Autodesk Fusion 360 part; units mm, degrees
note: some values were not read from the file. Set by a fixed rule: which sketch regions a step uses.
(part 8 of 10)
  spline S44 degree 5 poles (-2.127, 15.858) (-2.1276, 15.856) (-2.1289, 15.8519) (-2.1307, 15.8458) (-2.1332, 15.8377) (-2.1363, 15.8275) (-2.1394, 15.8174) (-2.1424, 15.8074) (-2.1454, 15.7973) (-2.1484, 15.7872) (-2.1514, 15.7772) (-2.1543, 15.7672) (-2.1573, 15.7572) (-2.1602, 15.7473) (-2.163, 15.7373) (-2.1659, 15.7274) (-2.1687, 15.7175) (-2.1715, 15.7076) (-2.1743, 15.6978) (-2.1771, 15.6879) (-2.1798, 15.6781) (-2.1825, 15.6683) (-2.1852, 15.6585) (-2.1879, 15.6488) (-2.1905, 15.6391) (-2.1931, 15.6294) (-2.1957, 15.6197) (-2.1983, 15.61) (-2.2008, 15.6004) (-2.2034, 15.5908) (-2.2059, 15.5812) (-2.2084, 15.5716) (-2.2108, 15.5621) (-2.2133, 15.5526) (-2.2157, 15.5431) (-2.2181, 15.5336) (-2.2204, 15.5241) (-2.2228, 15.5147) (-2.2251, 15.5053) (-2.2274, 15.4959) (-2.2297, 15.4866) (-2.232, 15.4772) (-2.2342, 15.4679) (-2.2364, 15.4586) (-2.2386, 15.4494) (-2.2408, 15.4402) (-2.2429, 15.431) (-2.2451, 15.4218) (-2.2472, 15.4126) (-2.2492, 15.4035) (-2.2513, 15.3944) (-2.2533, 15.3853) (-2.2554, 15.3762) (-2.2574, 15.3672) (-2.2593, 15.3582) (-2.2613, 15.3492) (-2.2632, 15.3403) (-2.2651, 15.3313) (-2.267, 15.3224) (-2.2689, 15.3136) (-2.2707, 15.3047) (-2.2726, 15.2959) (-2.2744, 15.2871) (-2.2761, 15.2784) (-2.2779, 15.2696) (-2.2796, 15.2609) (-2.2814, 15.2522) (-2.2831, 15.2436) (-2.2847, 15.2349) (-2.2864, 15.2263) (-2.288, 15.2178) (-2.2897, 15.2092) (-2.2913, 15.2007) (-2.2928, 15.1922) (-2.2944, 15.1838) (-2.2959, 15.1753) (-2.2974, 15.1669) (-2.2989, 15.1586) (-2.3004, 15.1502) (-2.3019, 15.1419) (-2.3033, 15.1336) (-2.3047, 15.1254) (-2.3061, 15.1172) (-2.3075, 15.109) (-2.3088, 15.1008) (-2.3102, 15.0927) (-2.3115, 15.0846) (-2.3128, 15.0765) (-2.3141, 15.0685) (-2.3153, 15.0605) (-2.3166, 15.0525) (-2.3178, 15.0445) (-2.319, 15.0366) (-2.3202, 15.0288) (-2.3213, 15.0209) (-2.3225, 15.0131) (-2.3236, 15.0053) (-2.3247, 14.9975) (-2.3258, 14.9898) (-2.3269, 14.9821) (-2.3279, 14.9745) (-2.329, 14.9669) (-2.33, 14.9593) (-2.331, 14.9517) (-2.332, 14.9442) (-2.3329, 14.9367) (-2.3339, 14.9292) (-2.3348, 14.9218) (-2.3357, 14.9144) (-2.3366, 14.9071) (-2.3375, 14.8998) (-2.3383, 14.8925) (-2.3391, 14.8852) (-2.34, 14.878) (-2.3408, 14.8708) (-2.3416, 14.8637) (-2.3423, 14.8566) (-2.3431, 14.8495) (-2.3438, 14.8425) (-2.3445, 14.8355) (-2.3452, 14.8285) (-2.3459, 14.8216) (-2.3466, 14.8147) (-2.3472, 14.8079) (-2.3479, 14.801) (-2.3485, 14.7943) (-2.3491, 14.7875) (-2.3497, 14.7808) (-2.3503, 14.7742) (-2.3508, 14.7675) (-2.3513, 14.7609) (-2.3519, 14.7544) (-2.3524, 14.7479) (-2.3529, 14.7414) (-2.3534, 14.735) (-2.3538, 14.7286) (-2.3543, 14.7222) (-2.3547, 14.7159) (-2.3551, 14.7097) (-2.3555, 14.7034) (-2.3559, 14.6972) (-2.3563, 14.6911) (-2.3567, 14.685) (-2.357, 14.6789) (-2.3574, 14.6729) (-2.3577, 14.6669) (-2.358, 14.6609) (-2.3583, 14.655) (-2.3586, 14.6492) (-2.3588, 14.6434) (-2.3591, 14.6376) (-2.3593, 14.6319) (-2.3596, 14.6262) (-2.3598, 14.6205) (-2.36, 14.6149) (-2.3602, 14.6094) (-2.3603, 14.6039) (-2.3605, 14.5984) (-2.3607, 14.593) (-2.3608, 14.5876) (-2.3609, 14.5823) (-2.3611, 14.577) (-2.3612, 14.5718) (-2.3613, 14.5666) (-2.3614, 14.5614) (-2.3614, 14.5563) (-2.3615, 14.5513) (-2.3616, 14.5463) (-2.3616, 14.5413) (-2.3616, 14.5364) (-2.3617, 14.5315) (-2.3617, 14.5267) (-2.3617, 14.5219) (-2.3617, 14.5172) (-2.3616, 14.5126) (-2.3616, 14.5079) (-2.3616, 14.5034) (-2.3616, 14.4989) (-2.3615, 14.4944) (-2.3614, 14.49) (-2.3614, 14.4856) (-2.3613, 14.4813) (-2.3612, 14.477) (-2.3611, 14.4728) (-2.361, 14.4687) (-2.3609, 14.4646) (-2.3608, 14.4605) (-2.3607, 14.4565) (-2.3606, 14.4526) (-2.3604, 14.4487) (-2.3603, 14.4449) (-2.3602, 14.4411) (-2.36, 14.4374) (-2.3599, 14.4337) (-2.3597, 14.4301) (-2.3595, 14.4265) (-2.3594, 14.423) (-2.3592, 14.4196) (-2.359, 14.4162) (-2.3588, 14.4129) (-2.3586, 14.4096) (-2.3584, 14.4064) (-2.3583, 14.4032) (-2.3581, 14.4001) (-2.3579, 14.3971) (-2.3577, 14.3941) (-2.3575, 14.3912) (-2.3572, 14.3884) (-2.357, 14.3856) (-2.3568, 14.3829) (-2.3566, 14.3802) (-2.3564, 14.3776) (-2.3562, 14.3751) (-2.356, 14.3726) (-2.3558, 14.3702) (-2.3556, 14.3679) (-2.3554, 14.3656) (-2.3551, 14.3634) (-2.3549, 14.3612) (-2.3547, 14.3591) (-2.3545, 14.3571) (-2.3543, 14.3552) (-2.3541, 14.3533) (-2.3539, 14.3515) (-2.3537, 14.3498) (-2.3536, 14.3481) (-2.3534, 14.3465) (-2.3532, 14.345) (-2.353, 14.3436) (-2.3529, 14.3422) (-2.3527, 14.3409) (-2.3525, 14.3397) (-2.3524, 14.3385) (-2.3522, 14.3374) (-2.3521, 14.3364) (-2.352, 14.3355) (-2.3519, 14.3346) (-2.3518, 14.3339) (-2.3517, 14.3332) (-2.3516, 14.3326) (-2.3515, 14.332) (-2.3514, 14.3317) (-2.3514, 14.3314) (-2.3514, 14.3313) (-2.3514, 14.3312) knots -1 -1 -1 -1 -1 -1 -0.99583333 -0.99166667 -0.9875 -0.98333333 -0.97916667 -0.975 -0.97083333 -0.96666667 -0.9625 -0.95833333 -0.95416667 -0.95 -0.94583333 -0.94166667 -0.9375 -0.93333333 -0.92916667 -0.925 -0.92083333 -0.91666667 -0.9125 -0.90833333 -0.90416667 -0.9 -0.89583333 -0.89166667 -0.8875 -0.88333333 -0.87916667 -0.875 -0.87083333 -0.86666667 -0.8625 -0.85833333 -0.85416667 -0.85 -0.84583333 -0.84166667 -0.8375 -0.83333333 -0.82916667 -0.825 -0.82083333 -0.81666667 -0.8125 -0.80833333 -0.80416667 -0.8 -0.79583333 -0.79166667 -0.7875 -0.78333333 -0.77916667 -0.775 -0.77083333 -0.76666667 -0.7625 -0.75833333 -0.75416667 -0.75 -0.74583333 -0.74166667 -0.7375 -0.73333333 -0.72916667 -0.725 -0.72083333 -0.71666667 -0.7125 -0.70833333 -0.70416667 -0.7 -0.69583333 -0.69166667 -0.6875 -0.68333333 -0.67916667 -0.675 -0.67083333 -0.66666667 -0.6625 -0.65833333 -0.65416667 -0.65 -0.64583333 -0.64166667 -0.6375 -0.63333333 -0.62916667 -0.625 -0.62083333 -0.61666667 -0.6125 -0.60833333 -0.60416667 -0.6 -0.59583333 -0.59166667 -0.5875 -0.58333333 -0.57916667 -0.575 -0.57083333 -0.56666667 -0.5625 -0.55833333 -0.55416667 -0.55 -0.54583333 -0.54166667 -0.5375 -0.53333333 -0.52916667 -0.525 -0.52083333 -0.51666667 -0.5125 -0.50833333 -0.50416667 -0.5 -0.49583333 -0.49166667 -0.4875 -0.48333333 -0.47916667 -0.475 -0.47083333 -0.46666667 -0.4625 -0.45833333 -0.45416667 -0.45 -0.44583333 -0.44166667 -0.4375 -0.43333333 -0.42916667 -0.425 -0.42083333 -0.41666667 -0.4125 -0.40833333 -0.40416667 -0.4 -0.39583333 -0.39166667 -0.3875 -0.38333333 -0.37916667 -0.375 -0.37083333 -0.36666667 -0.3625 -0.35833333 -0.35416667 -0.35 -0.34583333 -0.34166667 -0.3375 -0.33333333 -0.32916667 -0.325 -0.32083333 -0.31666667 -0.3125 -0.30833333 -0.30416667 -0.3 -0.29583333 -0.29166667 -0.2875 -0.28333333 -0.27916667 -0.275 -0.27083333 -0.26666667 -0.2625 -0.25833333 -0.25416667 -0.25 -0.24583333 -0.24166667 -0.2375 -0.23333333 -0.22916667 -0.225 -0.22083333 -0.21666667 -0.2125 -0.20833333 -0.20416667 -0.2 -0.19583333 -0.19166667 -0.1875 -0.18333333 -0.17916667 -0.175 -0.17083333 -0.16666667 -0.1625 -0.15833333 -0.15416667 -0.15 -0.14583333 -0.14166667 -0.1375 -0.13333333 -0.12916667 -0.125 -0.12083333 -0.11666667 -0.1125 -0.10833333 -0.10416667 -0.1 -0.09583333 -0.09166667 -0.0875 -0.08333333 -0.07916667 -0.075 -0.07083333 -0.06666667 -0.0625 -0.05833333 -0.05416667 -0.05 -0.04583333 -0.04166667 -0.0375 -0.03333333 -0.02916667 -0.025 -0.02083333 -0.01666667 -0.0125 -0.00833333 -0.00416667 0 0 0 0 0 0
  arc A51 (-11.5731, 7.4247) -> (-12.2165, 6.3102) centre (0, 0) ccw
  spline S45 degree 5 poles (-0.6796, 14.5069) (-0.6796, 14.507) (-0.6797, 14.5072) (-0.6797, 14.5074) (-0.6797, 14.5078) (-0.6797, 14.5083) (-0.6798, 14.5089) (-0.6798, 14.5096) (-0.6799, 14.5104) (-0.6799, 14.5112) (-0.68, 14.5122) (-0.6801, 14.5132) (-0.6802, 14.5143) (-0.6803, 14.5154) (-0.6804, 14.5167) (-0.6805, 14.518) (-0.6806, 14.5193) (-0.6807, 14.5208) (-0.6809, 14.5223) (-0.681, 14.5239) (-0.6812, 14.5256) (-0.6814, 14.5273) (-0.6815, 14.5291) (-0.6817, 14.531) (-0.6819, 14.5329) (-0.6822, 14.5349) (-0.6824, 14.537) (-0.6826, 14.5392) (-0.6829, 14.5414) (-0.6832, 14.5436) (-0.6834, 14.546) (-0.6837, 14.5484) (-0.684, 14.5508) (-0.6844, 14.5533) (-0.6847, 14.5559) (-0.685, 14.5586) (-0.6854, 14.5613) (-0.6858, 14.5641) (-0.6862, 14.5669) (-0.6866, 14.5698) (-0.687, 14.5727) (-0.6874, 14.5757) (-0.6879, 14.5788) (-0.6883, 14.5819) (-0.6888, 14.5851) (-0.6893, 14.5883) (-0.6898, 14.5916) (-0.6904, 14.595) (-0.6909, 14.5984) (-0.6915, 14.6018) (-0.6921, 14.6054) (-0.6926, 14.6089) (-0.6933, 14.6125) (-0.6939, 14.6162) (-0.6945, 14.6199) (-0.6952, 14.6237) (-0.6959, 14.6275) (-0.6966, 14.6314) (-0.6973, 14.6354) (-0.698, 14.6394) (-0.6988, 14.6434) (-0.6995, 14.6475) (-0.7003, 14.6516) (-0.7011, 14.6558) (-0.702, 14.66) (-0.7028, 14.6643) (-0.7037, 14.6686) (-0.7045, 14.673) (-0.7054, 14.6774) (-0.7064, 14.6819) (-0.7073, 14.6864) (-0.7082, 14.691) (-0.7092, 14.6956) (-0.7102, 14.7003) (-0.7112, 14.705) (-0.7123, 14.7097) (-0.7133, 14.7145) (-0.7144, 14.7194) (-0.7155, 14.7243) (-0.7166, 14.7292) (-0.7177, 14.7342) (-0.7189, 14.7392) (-0.7201, 14.7442) (-0.7213, 14.7493) (-0.7225, 14.7545) (-0.7237, 14.7597) (-0.725, 14.7649) (-0.7263, 14.7702) (-0.7276, 14.7755) (-0.7289, 14.7808) (-0.7302, 14.7862) (-0.7316, 14.7917) (-0.733, 14.7971) (-0.7344, 14.8027) (-0.7358, 14.8082) (-0.7372, 14.8138) (-0.7387, 14.8194) (-0.7402, 14.8251) (-0.7417, 14.8308) (-0.7433, 14.8366) (-0.7448, 14.8424) (-0.7464, 14.8482) (-0.748, 14.854) (-0.7496, 14.86) (-0.7513, 14.8659) (-0.7529, 14.8719) (-0.7546, 14.8779) (-0.7564, 14.8839) (-0.7581, 14.89) (-0.7599, 14.8961) (-0.7616, 14.9023) (-0.7634, 14.9085) (-0.7653, 14.9147) (-0.7671, 14.921) (-0.769, 14.9273) (-0.7709, 14.9336) (-0.7728, 14.94) (-0.7748, 14.9464) (-0.7767, 14.9528) (-0.7787, 14.9593) (-0.7807, 14.9658) (-0.7828, 14.9723) (-0.7848, 14.9789) (-0.7869, 14.9855) (-0.789, 14.9921) (-0.7912, 14.9987) (-0.7933, 15.0054) (-0.7955, 15.0122) (-0.7977, 15.0189) (-0.8, 15.0257) (-0.8022, 15.0325) (-0.8045, 15.0394) (-0.8068, 15.0463) (-0.8091, 15.0532) (-0.8115, 15.0601) (-0.8138, 15.0671) (-0.8162, 15.0741) (-0.8187, 15.0812) (-0.8211, 15.0882) (-0.8236, 15.0953) (-0.8261, 15.1025) (-0.8286, 15.1096) (-0.8311, 15.1168) (-0.8337, 15.124) (-0.8363, 15.1313) (-0.8389, 15.1385) (-0.8416, 15.1458) (-0.8442, 15.1531) (-0.8469, 15.1605) (-0.8497, 15.1679) (-0.8524, 15.1753) (-0.8552, 15.1827) (-0.858, 15.1902) (-0.8608, 15.1977) (-0.8636, 15.2052) (-0.8665, 15.2127) (-0.8694, 15.2203) (-0.8723, 15.2279) (-0.8753, 15.2355) (-0.8782, 15.2432) (-0.8812, 15.2509) (-0.8843, 15.2586) (-0.8873, 15.2663) (-0.8904, 15.274) (-0.8935, 15.2818) (-0.8966, 15.2896) (-0.8998, 15.2974) (-0.9029, 15.3053) (-0.9061, 15.3132) (-0.9094, 15.3211) (-0.9126, 15.329) (-0.9159, 15.3369) (-0.9192, 15.3449) (-0.9225, 15.3529) (-0.9259, 15.3609) (-0.9293, 15.369) (-0.9327, 15.377) (-0.9361, 15.3851) (-0.9396, 15.3932) (-0.9431, 15.4014) (-0.9466, 15.4095) (-0.9501, 15.4177) (-0.9537, 15.4259) (-0.9573, 15.4341) (-0.9609, 15.4424) (-0.9646, 15.4507) (-0.9682, 15.459) (-0.9719, 15.4673) (-0.9757, 15.4756) (-0.9794, 15.484) (-0.9832, 15.4923) (-0.987, 15.5007) (-0.9908, 15.5091) (-0.9947, 15.5176) (-0.9986, 15.526) (-1.0025, 15.5345) (-1.0064, 15.543) (-1.0104, 15.5515) (-1.0144, 15.5601) (-1.0184, 15.5686) (-1.0224, 15.5772) (-1.0265, 15.5858) (-1.0306, 15.5944) (-1.0347, 15.6031) (-1.0389, 15.6117) (-1.043, 15.6204) (-1.0472, 15.6291) (-1.0515, 15.6378) (-1.0557, 15.6466) (-1.06, 15.6553) (-1.0643, 15.6641) (-1.0687, 15.6729) (-1.073, 15.6817) (-1.0774, 15.6905) (-1.0818, 15.6993) (-1.0863, 15.7082) (-1.0907, 15.7171) (-1.0952, 15.726) (-1.0998, 15.7349) (-1.1043, 15.7438) (-1.1089, 15.7528) (-1.1135, 15.7617) (-1.1182, 15.7707) (-1.1228, 15.7797) (-1.1275, 15.7887) (-1.1322, 15.7977) (-1.137, 15.8068) (-1.1417, 15.8159) (-1.1465, 15.8249) (-1.1514, 15.834) (-1.1562, 15.8431) (-1.1611, 15.8523) (-1.166, 15.8614) (-1.1709, 15.8706) (-1.1759, 15.8797) (-1.1809, 15.8889) (-1.1859, 15.8981) (-1.1909, 15.9074) (-1.196, 15.9166) (-1.2011, 15.9258) (-1.2062, 15.9351) (-1.2104, 15.9425) (-1.2135, 15.9481) (-1.2155, 15.9518) (-1.2166, 15.9537) knots 0 0 0 0 0 0 0.00416667 0.00833333 0.0125 0.01666667 0.02083333 0.025 0.02916667 0.03333333 0.0375 0.04166667 0.04583333 0.05 0.05416667 0.05833333 0.0625 0.06666667 0.07083333 0.075 0.07916667 0.08333333 0.0875 0.09166667 0.09583333 0.1 0.10416667 0.10833333 0.1125 0.11666667 0.12083333 0.125 0.12916667 0.13333333 0.1375 0.14166667 0.14583333 0.15 0.15416667 0.15833333 0.1625 0.16666667 0.17083333 0.175 0.17916667 0.18333333 0.1875 0.19166667 0.19583333 0.2 0.20416667 0.20833333 0.2125 0.21666667 0.22083333 0.225 0.22916667 0.23333333 0.2375 0.24166667 0.24583333 0.25 0.25416667 0.25833333 0.2625 0.26666667 0.27083333 0.275 0.27916667 0.28333333 0.2875 0.29166667 0.29583333 0.3 0.30416667 0.30833333 0.3125 0.31666667 0.32083333 0.325 0.32916667 0.33333333 0.3375 0.34166667 0.34583333 0.35 0.35416667 0.35833333 0.3625 0.36666667 0.37083333 0.375 0.37916667 0.38333333 0.3875 0.39166667 0.39583333 0.4 0.40416667 0.40833333 0.4125 0.41666667 0.42083333 0.425 0.42916667 0.43333333 0.4375 0.44166667 0.44583333 0.45 0.45416667 0.45833333 0.4625 0.46666667 0.47083333 0.475 0.47916667 0.48333333 0.4875 0.49166667 0.49583333 0.5 0.50416667 0.50833333 0.5125 0.51666667 0.52083333 0.525 0.52916667 0.53333333 0.5375 0.54166667 0.54583333 0.55 0.55416667 0.55833333 0.5625 0.56666667 0.57083333 0.575 0.57916667 0.58333333 0.5875 0.59166667 0.59583333 0.6 0.60416667 0.60833333 0.6125 0.61666667 0.62083333 0.625 0.62916667 0.63333333 0.6375 0.64166667 0.64583333 0.65 0.65416667 0.65833333 0.6625 0.66666667 0.67083333 0.675 0.67916667 0.68333333 0.6875 0.69166667 0.69583333 0.7 0.70416667 0.70833333 0.7125 0.71666667 0.72083333 0.725 0.72916667 0.73333333 0.7375 0.74166667 0.74583333 0.75 0.75416667 0.75833333 0.7625 0.76666667 0.77083333 0.775 0.77916667 0.78333333 0.7875 0.79166667 0.79583333 0.8 0.80416667 0.80833333 0.8125 0.81666667 0.82083333 0.825 0.82916667 0.83333333 0.8375 0.84166667 0.84583333 0.85 0.85416667 0.85833333 0.8625 0.86666667 0.87083333 0.875 0.87916667 0.88333333 0.8875 0.89166667 0.89583333 0.9 0.90416667 0.90833333 0.9125 0.91666667 0.92083333 0.925 0.92916667 0.93333333 0.9375 0.94166667 0.94583333 0.95 0.95416667 0.95833333 0.9625 0.96666667 0.97083333 0.975 0.97916667 0.98333333 0.9875 0.99166667 0.99583333 1 1 1 1 1 1
  line L90 (0.6796, 14.5063) -> (0.6435, 13.7349)
  arc A52 (0.6435, 13.7349) -> (-0.6435, 13.7349) centre (0, 0) ccw
  arc A53 (-4.5069, 15.3521) -> (-5.3776, 15.0692) centre (0, 0) ccw
  line L91 (-2.3513, -14.3306) -> (-2.3514, -14.3312)
  spline S46 degree 5 poles (-2.3514, -14.3312) (-2.3514, -14.3313) (-2.3514, -14.3314) (-2.3514, -14.3317) (-2.3515, -14.332) (-2.3516, -14.3326) (-2.3517, -14.3332) (-2.3518, -14.3339) (-2.3519, -14.3346) (-2.352, -14.3355) (-2.3521, -14.3364) (-2.3522, -14.3374) (-2.3524, -14.3385) (-2.3525, -14.3397) (-2.3527, -14.3409) (-2.3529, -14.3422) (-2.353, -14.3436) (-2.3532, -14.345) (-2.3534, -14.3465) (-2.3536, -14.3481) (-2.3537, -14.3498) (-2.3539, -14.3515) (-2.3541, -14.3533) (-2.3543, -14.3552) (-2.3545, -14.3571) (-2.3547, -14.3591) (-2.3549, -14.3612) (-2.3551, -14.3634) (-2.3554, -14.3656) (-2.3556, -14.3679) (-2.3558, -14.3702) (-2.356, -14.3726) (-2.3562, -14.3751) (-2.3564, -14.3776) (-2.3566, -14.3802) (-2.3568, -14.3829) (-2.357, -14.3856) (-2.3572, -14.3884) (-2.3575, -14.3912) (-2.3577, -14.3941) (-2.3579, -14.3971) (-2.3581, -14.4001) (-2.3583, -14.4032) (-2.3584, -14.4064) (-2.3586, -14.4096) (-2.3588, -14.4129) (-2.359, -14.4162) (-2.3592, -14.4196) (-2.3594, -14.423) (-2.3595, -14.4265) (-2.3597, -14.4301) (-2.3599, -14.4337) (-2.36, -14.4374) (-2.3602, -14.4411) (-2.3603, -14.4449) (-2.3604, -14.4487) (-2.3606, -14.4526) (-2.3607, -14.4565) (-2.3608, -14.4605) (-2.3609, -14.4646) (-2.361, -14.4687) (-2.3611, -14.4728) (-2.3612, -14.477) (-2.3613, -14.4813) (-2.3614, -14.4856) (-2.3614, -14.49) (-2.3615, -14.4944) (-2.3616, -14.4989) (-2.3616, -14.5034) (-2.3616, -14.5079) (-2.3616, -14.5126) (-2.3617, -14.5172) (-2.3617, -14.5219) (-2.3617, -14.5267) (-2.3617, -14.5315) (-2.3616, -14.5364) (-2.3616, -14.5413) (-2.3616, -14.5463) (-2.3615, -14.5513) (-2.3614, -14.5563) (-2.3614, -14.5614) (-2.3613, -14.5666) (-2.3612, -14.5718) (-2.3611, -14.577) (-2.3609, -14.5823) (-2.3608, -14.5876) (-2.3607, -14.593) (-2.3605, -14.5984) (-2.3603, -14.6039) (-2.3602, -14.6094) (-2.36, -14.6149) (-2.3598, -14.6205) (-2.3596, -14.6262) (-2.3593, -14.6319) (-2.3591, -14.6376) (-2.3588, -14.6434) (-2.3586, -14.6492) (-2.3583, -14.655) (-2.358, -14.6609) (-2.3577, -14.6669) (-2.3574, -14.6729) (-2.357, -14.6789) (-2.3567, -14.685) (-2.3563, -14.6911) (-2.3559, -14.6972) (-2.3555, -14.7034) (-2.3551, -14.7097) (-2.3547, -14.7159) (-2.3543, -14.7222) (-2.3538, -14.7286) (-2.3534, -14.735) (-2.3529, -14.7414) (-2.3524, -14.7479) (-2.3519, -14.7544) (-2.3513, -14.7609) (-2.3508, -14.7675) (-2.3503, -14.7742) (-2.3497, -14.7808) (-2.3491, -14.7875) (-2.3485, -14.7943) (-2.3479, -14.801) (-2.3472, -14.8079) (-2.3466, -14.8147) (-2.3459, -14.8216) (-2.3452, -14.8285) (-2.3445, -14.8355) (-2.3438, -14.8425) (-2.3431, -14.8495) (-2.3423, -14.8566) (-2.3416, -14.8637) (-2.3408, -14.8708) (-2.34, -14.878) (-2.3391, -14.8852) (-2.3383, -14.8925) (-2.3375, -14.8998) (-2.3366, -14.9071) (-2.3357, -14.9144) (-2.3348, -14.9218) (-2.3339, -14.9292) (-2.3329, -14.9367) (-2.332, -14.9442) (-2.331, -14.9517) (-2.33, -14.9593) (-2.329, -14.9669) (-2.3279, -14.9745) (-2.3269, -14.9821) (-2.3258, -14.9898) (-2.3247, -14.9975) (-2.3236, -15.0053) (-2.3225, -15.0131) (-2.3213, -15.0209) (-2.3202, -15.0288) (-2.319, -15.0366) (-2.3178, -15.0445) (-2.3166, -15.0525) (-2.3153, -15.0605) (-2.3141, -15.0685) (-2.3128, -15.0765) (-2.3115, -15.0846) (-2.3102, -15.0927) (-2.3088, -15.1008) (-2.3075, -15.109) (-2.3061, -15.1172) (-2.3047, -15.1254) (-2.3033, -15.1336) (-2.3019, -15.1419) (-2.3004, -15.1502) (-2.2989, -15.1586) (-2.2974, -15.1669) (-2.2959, -15.1753) (-2.2944, -15.1838) (-2.2928, -15.1922) (-2.2913, -15.2007) (-2.2897, -15.2092) (-2.288, -15.2178) (-2.2864, -15.2263) (-2.2847, -15.2349) (-2.2831, -15.2436) (-2.2814, -15.2522) (-2.2796, -15.2609) (-2.2779, -15.2696) (-2.2761, -15.2784) (-2.2744, -15.2871) (-2.2726, -15.2959) (-2.2707, -15.3047) (-2.2689, -15.3136) (-2.267, -15.3224) (-2.2651, -15.3313) (-2.2632, -15.3403) (-2.2613, -15.3492) (-2.2593, -15.3582) (-2.2574, -15.3672) (-2.2554, -15.3762) (-2.2533, -15.3853) (-2.2513, -15.3944) (-2.2492, -15.4035) (-2.2472, -15.4126) (-2.2451, -15.4218) (-2.2429, -15.431) (-2.2408, -15.4402) (-2.2386, -15.4494) (-2.2364, -15.4586) (-2.2342, -15.4679) (-2.232, -15.4772) (-2.2297, -15.4866) (-2.2274, -15.4959) (-2.2251, -15.5053) (-2.2228, -15.5147) (-2.2204, -15.5241) (-2.2181, -15.5336) (-2.2157, -15.5431) (-2.2133, -15.5526) (-2.2108, -15.5621) (-2.2084, -15.5716) (-2.2059, -15.5812) (-2.2034, -15.5908) (-2.2008, -15.6004) (-2.1983, -15.61) (-2.1957, -15.6197) (-2.1931, -15.6294) (-2.1905, -15.6391) (-2.1879, -15.6488) (-2.1852, -15.6585) (-2.1825, -15.6683) (-2.1798, -15.6781) (-2.1771, -15.6879) (-2.1743, -15.6978) (-2.1715, -15.7076) (-2.1687, -15.7175) (-2.1659, -15.7274) (-2.163, -15.7373) (-2.1602, -15.7473) (-2.1573, -15.7572) (-2.1543, -15.7672) (-2.1514, -15.7772) (-2.1484, -15.7872) (-2.1454, -15.7973) (-2.1424, -15.8074) (-2.1394, -15.8174) (-2.1363, -15.8275) (-2.1332, -15.8377) (-2.1307, -15.8458) (-2.1289, -15.8519) (-2.1276, -15.856) (-2.127, -15.858) knots 0 0 0 0 0 0 0.00416667 0.00833333 0.0125 0.01666667 0.02083333 0.025 0.02916667 0.03333333 0.0375 0.04166667 0.04583333 0.05 0.05416667 0.05833333 0.0625 0.06666667 0.07083333 0.075 0.07916667 0.08333333 0.0875 0.09166667 0.09583333 0.1 0.10416667 0.10833333 0.1125 0.11666667 0.12083333 0.125 0.12916667 0.13333333 0.1375 0.14166667 0.14583333 0.15 0.15416667 0.15833333 0.1625 0.16666667 0.17083333 0.175 0.17916667 0.18333333 0.1875 0.19166667 0.19583333 0.2 0.20416667 0.20833333 0.2125 0.21666667 0.22083333 0.225 0.22916667 0.23333333 0.2375 0.24166667 0.24583333 0.25 0.25416667 0.25833333 0.2625 0.26666667 0.27083333 0.275 0.27916667 0.28333333 0.2875 0.29166667 0.29583333 0.3 0.30416667 0.30833333 0.3125 0.31666667 0.32083333 0.325 0.32916667 0.33333333 0.3375 0.34166667 0.34583333 0.35 0.35416667 0.35833333 0.3625 0.36666667 0.37083333 0.375 0.37916667 0.38333333 0.3875 0.39166667 0.39583333 0.4 0.40416667 0.40833333 0.4125 0.41666667 0.42083333 0.425 0.42916667 0.43333333 0.4375 0.44166667 0.44583333 0.45 0.45416667 0.45833333 0.4625 0.46666667 0.47083333 0.475 0.47916667 0.48333333 0.4875 0.49166667 0.49583333 0.5 0.50416667 0.50833333 0.5125 0.51666667 0.52083333 0.525 0.52916667 0.53333333 0.5375 0.54166667 0.54583333 0.55 0.55416667 0.55833333 0.5625 0.56666667 0.57083333 0.575 0.57916667 0.58333333 0.5875 0.59166667 0.59583333 0.6 0.60416667 0.60833333 0.6125 0.61666667 0.62083333 0.625 0.62916667 0.63333333 0.6375 0.64166667 0.64583333 0.65 0.65416667 0.65833333 0.6625 0.66666667 0.67083333 0.675 0.67916667 0.68333333 0.6875 0.69166667 0.69583333 0.7 0.70416667 0.70833333 0.7125 0.71666667 0.72083333 0.725 0.72916667 0.73333333 0.7375 0.74166667 0.74583333 0.75 0.75416667 0.75833333 0.7625 0.76666667 0.77083333 0.775 0.77916667 0.78333333 0.7875 0.79166667 0.79583333 0.8 0.80416667 0.80833333 0.8125 0.81666667 0.82083333 0.825 0.82916667 0.83333333 0.8375 0.84166667 0.84583333 0.85 0.85416667 0.85833333 0.8625 0.86666667 0.87083333 0.875 0.87916667 0.88333333 0.8875 0.89166667 0.89583333 0.9 0.90416667 0.90833333 0.9125 0.91666667 0.92083333 0.925 0.92916667 0.93333333 0.9375 0.94166667 0.94583333 0.95 0.95416667 0.95833333 0.9625 0.96666667 0.97083333 0.975 0.97916667 0.98333333 0.9875 0.99166667 0.99583333 1 1 1 1 1 1
  arc A54 (-3.4851, -13.301) -> (-2.2262, -13.5686) centre (0, 0) ccw
  spline S47 degree 5 poles (1.2166, 15.9537) (1.2155, 15.9518) (1.2135, 15.9481) (1.2104, 15.9425) (1.2062, 15.9351) (1.2011, 15.9258) (1.196, 15.9166) (1.1909, 15.9074) (1.1859, 15.8981) (1.1809, 15.8889) (1.1759, 15.8797) (1.1709, 15.8706) (1.166, 15.8614) (1.1611, 15.8523) (1.1562, 15.8431) (1.1514, 15.834) (1.1465, 15.8249) (1.1417, 15.8159) (1.137, 15.8068) (1.1322, 15.7977) (1.1275, 15.7887) (1.1228, 15.7797) (1.1182, 15.7707) (1.1135, 15.7617) (1.1089, 15.7528) (1.1043, 15.7438) (1.0998, 15.7349) (1.0952, 15.726) (1.0907, 15.7171) (1.0863, 15.7082) (1.0818, 15.6993) (1.0774, 15.6905) (1.073, 15.6817) (1.0687, 15.6729) (1.0643, 15.6641) (1.06, 15.6553) (1.0557, 15.6466) (1.0515, 15.6378) (1.0472, 15.6291) (1.043, 15.6204) (1.0389, 15.6117) (1.0347, 15.6031) (1.0306, 15.5944) (1.0265, 15.5858) (1.0224, 15.5772) (1.0184, 15.5686) (1.0144, 15.5601) (1.0104, 15.5515) (1.0064, 15.543) (1.0025, 15.5345) (0.9986, 15.526) (0.9947, 15.5176) (0.9908, 15.5091) (0.987, 15.5007) (0.9832, 15.4923) (0.9794, 15.484) (0.9757, 15.4756) (0.9719, 15.4673) (0.9682, 15.459) (0.9646, 15.4507) (0.9609, 15.4424) (0.9573, 15.4341) (0.9537, 15.4259) (0.9501, 15.4177) (0.9466, 15.4095) (0.9431, 15.4014) (0.9396, 15.3932) (0.9361, 15.3851) (0.9327, 15.377) (0.9293, 15.369) (0.9259, 15.3609) (0.9225, 15.3529) (0.9192, 15.3449) (0.9159, 15.3369) (0.9126, 15.329) (0.9094, 15.3211) (0.9061, 15.3132) (0.9029, 15.3053) (0.8998, 15.2974) (0.8966, 15.2896) (0.8935, 15.2818) (0.8904, 15.274) (0.8873, 15.2663) (0.8843, 15.2586) (0.8812, 15.2509) (0.8782, 15.2432) (0.8753, 15.2355) (0.8723, 15.2279) (0.8694, 15.2203) (0.8665, 15.2127) (0.8636, 15.2052) (0.8608, 15.1977) (0.858, 15.1902) (0.8552, 15.1827) (0.8524, 15.1753) (0.8497, 15.1679) (0.8469, 15.1605) (0.8442, 15.1531) (0.8416, 15.1458) (0.8389, 15.1385) (0.8363, 15.1313) (0.8337, 15.124) (0.8311, 15.1168) (0.8286, 15.1096) (0.8261, 15.1025) (0.8236, 15.0953) (0.8211, 15.0882) (0.8187, 15.0812) (0.8162, 15.0741) (0.8138, 15.0671) (0.8115, 15.0601) (0.8091, 15.0532) (0.8068, 15.0463) (0.8045, 15.0394) (0.8022, 15.0325) (0.8, 15.0257) (0.7977, 15.0189) (0.7955, 15.0122) (0.7933, 15.0054) (0.7912, 14.9987) (0.789, 14.9921) (0.7869, 14.9855) (0.7848, 14.9789) (0.7828, 14.9723) (0.7807, 14.9658) (0.7787, 14.9593) (0.7767, 14.9528) (0.7748, 14.9464) (0.7728, 14.94) (0.7709, 14.9336) (0.769, 14.9273) (0.7671, 14.921) (0.7653, 14.9147) (0.7634, 14.9085) (0.7616, 14.9023) (0.7599, 14.8961) (0.7581, 14.89) (0.7564, 14.8839) (0.7546, 14.8779) (0.7529, 14.8719) (0.7513, 14.8659) (0.7496, 14.86) (0.748, 14.854) (0.7464, 14.8482) (0.7448, 14.8424) (0.7433, 14.8366) (0.7417, 14.8308) (0.7402, 14.8251) (0.7387, 14.8194) (0.7372, 14.8138) (0.7358, 14.8082) (0.7344, 14.8027) (0.733, 14.7971) (0.7316, 14.7917) (0.7302, 14.7862) (0.7289, 14.7808) (0.7276, 14.7755) (0.7263, 14.7702) (0.725, 14.7649) (0.7237, 14.7597) (0.7225, 14.7545) (0.7213, 14.7493) (0.7201, 14.7442) (0.7189, 14.7392) (0.7177, 14.7342) (0.7166, 14.7292) (0.7155, 14.7243) (0.7144, 14.7194) (0.7133, 14.7145) (0.7123, 14.7097) (0.7112, 14.705) (0.7102, 14.7003) (0.7092, 14.6956) (0.7082, 14.691) (0.7073, 14.6864) (0.7064, 14.6819) (0.7054, 14.6774) (0.7045, 14.673) (0.7037, 14.6686) (0.7028, 14.6643) (0.702, 14.66) (0.7011, 14.6558) (0.7003, 14.6516) (0.6995, 14.6475) (0.6988, 14.6434) (0.698, 14.6394) (0.6973, 14.6354) (0.6966, 14.6314) (0.6959, 14.6275) (0.6952, 14.6237) (0.6945, 14.6199) (0.6939, 14.6162) (0.6933, 14.6125) (0.6926, 14.6089) (0.6921, 14.6054) (0.6915, 14.6018) (0.6909, 14.5984) (0.6904, 14.595) (0.6898, 14.5916) (0.6893, 14.5883) (0.6888, 14.5851) (0.6883, 14.5819) (0.6879, 14.5788) (0.6874, 14.5757) (0.687, 14.5727) (0.6866, 14.5698) (0.6862, 14.5669) (0.6858, 14.5641) (0.6854, 14.5613) (0.685, 14.5586) (0.6847, 14.5559) (0.6844, 14.5533) (0.684, 14.5508) (0.6837, 14.5484) (0.6834, 14.546) (0.6832, 14.5436) (0.6829, 14.5414) (0.6826, 14.5392) (0.6824, 14.537) (0.6822, 14.5349) (0.6819, 14.5329) (0.6817, 14.531) (0.6815, 14.5291) (0.6814, 14.5273) (0.6812, 14.5256) (0.681, 14.5239) (0.6809, 14.5223) (0.6807, 14.5208) (0.6806, 14.5193) (0.6805, 14.518) (0.6804, 14.5167) (0.6803, 14.5154) (0.6802, 14.5143) (0.6801, 14.5132) (0.68, 14.5122) (0.6799, 14.5112) (0.6799, 14.5104) (0.6798, 14.5096) (0.6798, 14.5089) (0.6797, 14.5083) (0.6797, 14.5078) (0.6797, 14.5074) (0.6797, 14.5072) (0.6796, 14.507) (0.6796, 14.5069) knots -1 -1 -1 -1 -1 -1 -0.99583333 -0.99166667 -0.9875 -0.98333333 -0.97916667 -0.975 -0.97083333 -0.96666667 -0.9625 -0.95833333 -0.95416667 -0.95 -0.94583333 -0.94166667 -0.9375 -0.93333333 -0.92916667 -0.925 -0.92083333 -0.91666667 -0.9125 -0.90833333 -0.90416667 -0.9 -0.89583333 -0.89166667 -0.8875 -0.88333333 -0.87916667 -0.875 -0.87083333 -0.86666667 -0.8625 -0.85833333 -0.85416667 -0.85 -0.84583333 -0.84166667 -0.8375 -0.83333333 -0.82916667 -0.825 -0.82083333 -0.81666667 -0.8125 -0.80833333 -0.80416667 -0.8 -0.79583333 -0.79166667 -0.7875 -0.78333333 -0.77916667 -0.775 -0.77083333 -0.76666667 -0.7625 -0.75833333 -0.75416667 -0.75 -0.74583333 -0.74166667 -0.7375 -0.73333333 -0.72916667 -0.725 -0.72083333 -0.71666667 -0.7125 -0.70833333 -0.70416667 -0.7 -0.69583333 -0.69166667 -0.6875 -0.68333333 -0.67916667 -0.675 -0.67083333 -0.66666667 -0.6625 -0.65833333 -0.65416667 -0.65 -0.64583333 -0.64166667 -0.6375 -0.63333333 -0.62916667 -0.625 -0.62083333 -0.61666667 -0.6125 -0.60833333 -0.60416667 -0.6 -0.59583333 -0.59166667 -0.5875 -0.58333333 -0.57916667 -0.575 -0.57083333 -0.56666667 -0.5625 -0.55833333 -0.55416667 -0.55 -0.54583333 -0.54166667 -0.5375 -0.53333333 -0.52916667 -0.525 -0.52083333 -0.51666667 -0.5125 -0.50833333 -0.50416667 -0.5 -0.49583333 -0.49166667 -0.4875 -0.48333333 -0.47916667 -0.475 -0.47083333 -0.46666667 -0.4625 -0.45833333 -0.45416667 -0.45 -0.44583333 -0.44166667 -0.4375 -0.43333333 -0.42916667 -0.425 -0.42083333 -0.41666667 -0.4125 -0.40833333 -0.40416667 -0.4 -0.39583333 -0.39166667 -0.3875 -0.38333333 -0.37916667 -0.375 -0.37083333 -0.36666667 -0.3625 -0.35833333 -0.35416667 -0.35 -0.34583333 -0.34166667 -0.3375 -0.33333333 -0.32916667 -0.325 -0.32083333 -0.31666667 -0.3125 -0.30833333 -0.30416667 -0.3 -0.29583333 -0.29166667 -0.2875 -0.28333333 -0.27916667 -0.275 -0.27083333 -0.26666667 -0.2625 -0.25833333 -0.25416667 -0.25 -0.24583333 -0.24166667 -0.2375 -0.23333333 -0.22916667 -0.225 -0.22083333 -0.21666667 -0.2125 -0.20833333 -0.20416667 -0.2 -0.19583333 -0.19166667 -0.1875 -0.18333333 -0.17916667 -0.175 -0.17083333 -0.16666667 -0.1625 -0.15833333 -0.15416667 -0.15 -0.14583333 -0.14166667 -0.1375 -0.13333333 -0.12916667 -0.125 -0.12083333 -0.11666667 -0.1125 -0.10833333 -0.10416667 -0.1 -0.09583333 -0.09166667 -0.0875 -0.08333333 -0.07916667 -0.075 -0.07083333 -0.06666667 -0.0625 -0.05833333 -0.05416667 -0.05 -0.04583333 -0.04166667 -0.0375 -0.03333333 -0.02916667 -0.025 -0.02083333 -0.01666667 -0.0125 -0.00833333 -0.00416667 0 0 0 0 0 0
  arc A55 (-15.5488, 3.7729) -> (-15.7391, 2.8775) centre (0, 0) ccw
  line L92 (-14.3564, 2.1923) -> (-14.3558, 2.1922)
  line L93 (-2.2262, -13.5686) -> (-2.3513, -14.3306)
  line L94 (-14.3558, 2.1922) -> (-13.5924, 2.0756)
  line L95 (-12.223, 7.8417) -> (-11.5731, 7.4247)
  line L96 (-13.2615, 3.6324) -> (-14.0063, 3.8363)
  arc A56 (-5.3776, -15.0692) -> (-4.5069, -15.3521) centre (0, 0) ccw
  spline S48 degree 5 poles (-14.4985, 0.8405) (-14.4986, 0.8405) (-14.4987, 0.8405) (-14.499, 0.8405) (-14.4993, 0.8405) (-14.4999, 0.8405) (-14.5005, 0.8406) (-14.5012, 0.8406) (-14.502, 0.8406) (-14.5028, 0.8406) (-14.5037, 0.8407) (-14.5048, 0.8407) (-14.5058, 0.8407) (-14.507, 0.8407) (-14.5082, 0.8408) (-14.5096, 0.8408) (-14.5109, 0.8408) (-14.5124, 0.8408) (-14.5139, 0.8409) (-14.5155, 0.8409) (-14.5172, 0.8409) (-14.519, 0.8409) (-14.5208, 0.8409) (-14.5226, 0.8409) (-14.5246, 0.8409) (-14.5266, 0.8409) (-14.5287, 0.8409) (-14.5309, 0.8409) (-14.5331, 0.8408) (-14.5354, 0.8408) (-14.5377, 0.8408) (-14.5401, 0.8407) (-14.5426, 0.8407) (-14.5452, 0.8406) (-14.5478, 0.8406) (-14.5504, 0.8405) (-14.5532, 0.8404) (-14.556, 0.8403) (-14.5588, 0.8402) (-14.5617, 0.8401) (-14.5647, 0.84) (-14.5677, 0.8399) (-14.5708, 0.8398) (-14.574, 0.8396) (-14.5772, 0.8395) (-14.5805, 0.8393) (-14.5838, 0.8392) (-14.5872, 0.839) (-14.5906, 0.8388) (-14.5941, 0.8386) (-14.5977, 0.8384) (-14.6013, 0.8382) (-14.605, 0.838) (-14.6087, 0.8377) (-14.6124, 0.8375) (-14.6163, 0.8372) (-14.6202, 0.8369) (-14.6241, 0.8366) (-14.6281, 0.8363) (-14.6321, 0.836) (-14.6362, 0.8357) (-14.6404, 0.8354) (-14.6446, 0.835) (-14.6488, 0.8347) (-14.6531, 0.8343) (-14.6574, 0.8339) (-14.6618, 0.8335) (-14.6663, 0.8331) (-14.6708, 0.8326) (-14.6753, 0.8322) (-14.6799, 0.8317) (-14.6846, 0.8313) (-14.6893, 0.8308) (-14.694, 0.8303) (-14.6988, 0.8298) (-14.7036, 0.8292) (-14.7085, 0.8287) (-14.7134, 0.8281) (-14.7184, 0.8275) (-14.7234, 0.8269) (-14.7285, 0.8263) (-14.7336, 0.8257) (-14.7387, 0.8251) (-14.7439, 0.8244) (-14.7492, 0.8237) (-14.7545, 0.8231) (-14.7598, 0.8224) (-14.7652, 0.8216) (-14.7706, 0.8209) (-14.7761, 0.8201) (-14.7816, 0.8194) (-14.7871, 0.8186) (-14.7927, 0.8178) (-14.7983, 0.817) (-14.804, 0.8161) (-14.8097, 0.8153) (-14.8155, 0.8144) (-14.8213, 0.8135) (-14.8271, 0.8126) (-14.833, 0.8117) (-14.8389, 0.8107) (-14.8449, 0.8097) (-14.8509, 0.8088) (-14.8569, 0.8078) (-14.863, 0.8067) (-14.8691, 0.8057) (-14.8753, 0.8047) (-14.8814, 0.8036) (-14.8877, 0.8025) (-14.8939, 0.8014) (-14.9003, 0.8002) (-14.9066, 0.7991) (-14.913, 0.7979) (-14.9194, 0.7967) (-14.9259, 0.7955) (-14.9324, 0.7943) (-14.9389, 0.7931) (-14.9455, 0.7918) (-14.9521, 0.7905) (-14.9587, 0.7892) (-14.9654, 0.7879) (-14.9721, 0.7865) (-14.9788, 0.7852) (-14.9856, 0.7838) (-14.9924, 0.7824) (-14.9993, 0.781) (-15.0062, 0.7795) (-15.0131, 0.778) (-15.02, 0.7766) (-15.027, 0.775) (-15.0341, 0.7735) (-15.0411, 0.772) (-15.0482, 0.7704) (-15.0553, 0.7688) (-15.0625, 0.7672) (-15.0697, 0.7656) (-15.0769, 0.7639) (-15.0841, 0.7622) (-15.0914, 0.7605) (-15.0987, 0.7588) (-15.1061, 0.7571) (-15.1135, 0.7553) (-15.1209, 0.7535) (-15.1283, 0.7517) (-15.1358, 0.7499) (-15.1433, 0.7481) (-15.1508, 0.7462) (-15.1584, 0.7443) (-15.166, 0.7424) (-15.1736, 0.7405) (-15.1813, 0.7385) (-15.1889, 0.7365) (-15.1967, 0.7345) (-15.2044, 0.7325) (-15.2122, 0.7305) (-15.22, 0.7284) (-15.2278, 0.7263) (-15.2357, 0.7242) (-15.2436, 0.7221) (-15.2515, 0.7199) (-15.2594, 0.7177) (-15.2674, 0.7155) (-15.2754, 0.7133) (-15.2834, 0.7111) (-15.2915, 0.7088) (-15.2996, 0.7065) (-15.3077, 0.7042) (-15.3158, 0.7018) (-15.324, 0.6995) (-15.3322, 0.6971) (-15.3404, 0.6947) (-15.3487, 0.6923) (-15.3569, 0.6898) (-15.3652, 0.6873) (-15.3736, 0.6848) (-15.3819, 0.6823) (-15.3903, 0.6797) (-15.3987, 0.6772) (-15.4071, 0.6746) (-15.4156, 0.672) (-15.4241, 0.6693) (-15.4326, 0.6667) (-15.4411, 0.664) (-15.4497, 0.6613) (-15.4582, 0.6585) (-15.4668, 0.6558) (-15.4755, 0.653) (-15.4841, 0.6502) (-15.4928, 0.6473) (-15.5015, 0.6445) (-15.5102, 0.6416) (-15.519, 0.6387) (-15.5278, 0.6358) (-15.5365, 0.6328) (-15.5454, 0.6298) (-15.5542, 0.6268) (-15.5631, 0.6238) (-15.572, 0.6207) (-15.5809, 0.6177) (-15.5898, 0.6146) (-15.5988, 0.6114) (-15.6077, 0.6083) (-15.6167, 0.6051) (-15.6258, 0.6019) (-15.6348, 0.5987) (-15.6439, 0.5955) (-15.653, 0.5922) (-15.6621, 0.5889) (-15.6712, 0.5856) (-15.6803, 0.5822) (-15.6895, 0.5789) (-15.6987, 0.5755) (-15.7079, 0.572) (-15.7172, 0.5686) (-15.7264, 0.5651) (-15.7357, 0.5616) (-15.745, 0.5581) (-15.7543, 0.5546) (-15.7636, 0.551) (-15.773, 0.5474) (-15.7824, 0.5438) (-15.7918, 0.5401) (-15.8012, 0.5365) (-15.8106, 0.5328) (-15.8201, 0.529) (-15.8295, 0.5253) (-15.839, 0.5215) (-15.8486, 0.5177) (-15.8581, 0.5139) (-15.8676, 0.5101) (-15.8772, 0.5062) (-15.8868, 0.5023) (-15.8964, 0.4984) (-15.906, 0.4944) (-15.9157, 0.4904) (-15.9253, 0.4864) (-15.935, 0.4824) (-15.9447, 0.4784) (-15.9544, 0.4743) (-15.9641, 0.4702) (-15.9739, 0.466) (-15.9817, 0.4627) (-15.9876, 0.4602) (-15.9915, 0.4585) (-15.9935, 0.4577) knots 0 0 0 0 0 0 0.00416667 0.00833333 0.0125 0.01666667 0.02083333 0.025 0.02916667 0.03333333 0.0375 0.04166667 0.04583333 0.05 0.05416667 0.05833333 0.0625 0.06666667 0.07083333 0.075 0.07916667 0.08333333 0.0875 0.09166667 0.09583333 0.1 0.10416667 0.10833333 0.1125 0.11666667 0.12083333 0.125 0.12916667 0.13333333 0.1375 0.14166667 0.14583333 0.15 0.15416667 0.15833333 0.1625 0.16666667 0.17083333 0.175 0.17916667 0.18333333 0.1875 0.19166667 0.19583333 0.2 0.20416667 0.20833333 0.2125 0.21666667 0.22083333 0.225 0.22916667 0.23333333 0.2375 0.24166667 0.24583333 0.25 0.25416667 0.25833333 0.2625 0.26666667 0.27083333 0.275 0.27916667 0.28333333 0.2875 0.29166667 0.29583333 0.3 0.30416667 0.30833333 0.3125 0.31666667 0.32083333 0.325 0.32916667 0.33333333 0.3375 0.34166667 0.34583333 0.35 0.35416667 0.35833333 0.3625 0.36666667 0.37083333 0.375 0.37916667 0.38333333 0.3875 0.39166667 0.39583333 0.4 0.40416667 0.40833333 0.4125 0.41666667 0.42083333 0.425 0.42916667 0.43333333 0.4375 0.44166667 0.44583333 0.45 0.45416667 0.45833333 0.4625 0.46666667 0.47083333 0.475 0.47916667 0.48333333 0.4875 0.49166667 0.49583333 0.5 0.50416667 0.50833333 0.5125 0.51666667 0.52083333 0.525 0.52916667 0.53333333 0.5375 0.54166667 0.54583333 0.55 0.55416667 0.55833333 0.5625 0.56666667 0.57083333 0.575 0.57916667 0.58333333 0.5875 0.59166667 0.59583333 0.6 0.60416667 0.60833333 0.6125 0.61666667 0.62083333 0.625 0.62916667 0.63333333 0.6375 0.64166667 0.64583333 0.65 0.65416667 0.65833333 0.6625 0.66666667 0.67083333 0.675 0.67916667 0.68333333 0.6875 0.69166667 0.69583333 0.7 0.70416667 0.70833333 0.7125 0.71666667 0.72083333 0.725 0.72916667 0.73333333 0.7375 0.74166667 0.74583333 0.75 0.75416667 0.75833333 0.7625 0.76666667 0.77083333 0.775 0.77916667 0.78333333 0.7875 0.79166667 0.79583333 0.8 0.80416667 0.80833333 0.8125 0.81666667 0.82083333 0.825 0.82916667 0.83333333 0.8375 0.84166667 0.84583333 0.85 0.85416667 0.85833333 0.8625 0.86666667 0.87083333 0.875 0.87916667 0.88333333 0.8875 0.89166667 0.89583333 0.9 0.90416667 0.90833333 0.9125 0.91666667 0.92083333 0.925 0.92916667 0.93333333 0.9375 0.94166667 0.94583333 0.95 0.95416667 0.95833333 0.9625 0.96666667 0.97083333 0.975 0.97916667 0.98333333 0.9875 0.99166667 0.99583333 1 1 1 1 1 1
  line L97 (-0.6796, -14.5063) -> (-0.6435, -13.7349)
  arc A57 (-6.1743, -12.2858) -> (-4.9987, -12.8092) centre (0, 0) ccw
  line L98 (-12.2236, 7.8421) -> (-12.223, 7.8417)
  arc A58 (-2.127, -15.858) -> (-1.2166, -15.9537) centre (0, 0) ccw
  spline S49 degree 5 poles (2.3514, 14.3312) (2.3514, 14.3313) (2.3514, 14.3314) (2.3514, 14.3317) (2.3515, 14.332) (2.3516, 14.3326) (2.3517, 14.3332) (2.3518, 14.3339) (2.3519, 14.3346) (2.352, 14.3355) (2.3521, 14.3364) (2.3522, 14.3374) (2.3524, 14.3385) (2.3525, 14.3397) (2.3527, 14.3409) (2.3529, 14.3422) (2.353, 14.3436) (2.3532, 14.345) (2.3534, 14.3465) (2.3536, 14.3481) (2.3537, 14.3498) (2.3539, 14.3515) (2.3541, 14.3533) (2.3543, 14.3552) (2.3545, 14.3571) (2.3547, 14.3591) (2.3549, 14.3612) (2.3551, 14.3634) (2.3554, 14.3656) (2.3556, 14.3679) (2.3558, 14.3702) (2.356, 14.3726) (2.3562, 14.3751) (2.3564, 14.3776) (2.3566, 14.3802) (2.3568, 14.3829) (2.357, 14.3856) (2.3572, 14.3884) (2.3575, 14.3912) (2.3577, 14.3941) (2.3579, 14.3971) (2.3581, 14.4001) (2.3583, 14.4032) (2.3584, 14.4064) (2.3586, 14.4096) (2.3588, 14.4129) (2.359, 14.4162) (2.3592, 14.4196) (2.3594, 14.423) (2.3595, 14.4265) (2.3597, 14.4301) (2.3599, 14.4337) (2.36, 14.4374) (2.3602, 14.4411) (2.3603, 14.4449) (2.3604, 14.4487) (2.3606, 14.4526) (2.3607, 14.4565) (2.3608, 14.4605) (2.3609, 14.4646) (2.361, 14.4687) (2.3611, 14.4728) (2.3612, 14.477) (2.3613, 14.4813) (2.3614, 14.4856) (2.3614, 14.49) (2.3615, 14.4944) (2.3616, 14.4989) (2.3616, 14.5034) (2.3616, 14.5079) (2.3616, 14.5126) (2.3617, 14.5172) (2.3617, 14.5219) (2.3617, 14.5267) (2.3617, 14.5315) (2.3616, 14.5364) (2.3616, 14.5413) (2.3616, 14.5463) (2.3615, 14.5513) (2.3614, 14.5563) (2.3614, 14.5614) (2.3613, 14.5666) (2.3612, 14.5718) (2.3611, 14.577) (2.3609, 14.5823) (2.3608, 14.5876) (2.3607, 14.593) (2.3605, 14.5984) (2.3603, 14.6039) (2.3602, 14.6094) (2.36, 14.6149) (2.3598, 14.6205) (2.3596, 14.6262) (2.3593, 14.6319) (2.3591, 14.6376) (2.3588, 14.6434) (2.3586, 14.6492) (2.3583, 14.655) (2.358, 14.6609) (2.3577, 14.6669) (2.3574, 14.6729) (2.357, 14.6789) (2.3567, 14.685) (2.3563, 14.6911) (2.3559, 14.6972) (2.3555, 14.7034) (2.3551, 14.7097) (2.3547, 14.7159) (2.3543, 14.7222) (2.3538, 14.7286) (2.3534, 14.735) (2.3529, 14.7414) (2.3524, 14.7479) (2.3519, 14.7544) (2.3513, 14.7609) (2.3508, 14.7675) (2.3503, 14.7742) (2.3497, 14.7808) (2.3491, 14.7875) (2.3485, 14.7943) (2.3479, 14.801) (2.3472, 14.8079) (2.3466, 14.8147) (2.3459, 14.8216) (2.3452, 14.8285) (2.3445, 14.8355) (2.3438, 14.8425) (2.3431, 14.8495) (2.3423, 14.8566) (2.3416, 14.8637) (2.3408, 14.8708) (2.34, 14.878) (2.3391, 14.8852) (2.3383, 14.8925) (2.3375, 14.8998) (2.3366, 14.9071) (2.3357, 14.9144) (2.3348, 14.9218) (2.3339, 14.9292) (2.3329, 14.9367) (2.332, 14.9442) (2.331, 14.9517) (2.33, 14.9593) (2.329, 14.9669) (2.3279, 14.9745) (2.3269, 14.9821) (2.3258, 14.9898) (2.3247, 14.9975) (2.3236, 15.0053) (2.3225, 15.0131) (2.3213, 15.0209) (2.3202, 15.0288) (2.319, 15.0366) (2.3178, 15.0445) (2.3166, 15.0525) (2.3153, 15.0605) (2.3141, 15.0685) (2.3128, 15.0765) (2.3115, 15.0846) (2.3102, 15.0927) (2.3088, 15.1008) (2.3075, 15.109) (2.3061, 15.1172) (2.3047, 15.1254) (2.3033, 15.1336) (2.3019, 15.1419) (2.3004, 15.1502) (2.2989, 15.1586) (2.2974, 15.1669) (2.2959, 15.1753) (2.2944, 15.1838) (2.2928, 15.1922) (2.2913, 15.2007) (2.2897, 15.2092) (2.288, 15.2178) (2.2864, 15.2263) (2.2847, 15.2349) (2.2831, 15.2436) (2.2814, 15.2522) (2.2796, 15.2609) (2.2779, 15.2696) (2.2761, 15.2784) (2.2744, 15.2871) (2.2726, 15.2959) (2.2707, 15.3047) (2.2689, 15.3136) (2.267, 15.3224) (2.2651, 15.3313) (2.2632, 15.3403) (2.2613, 15.3492) (2.2593, 15.3582) (2.2574, 15.3672) (2.2554, 15.3762) (2.2533, 15.3853) (2.2513, 15.3944) (2.2492, 15.4035) (2.2472, 15.4126) (2.2451, 15.4218) (2.2429, 15.431) (2.2408, 15.4402) (2.2386, 15.4494) (2.2364, 15.4586) (2.2342, 15.4679) (2.232, 15.4772) (2.2297, 15.4866) (2.2274, 15.4959) (2.2251, 15.5053) (2.2228, 15.5147) (2.2204, 15.5241) (2.2181, 15.5336) (2.2157, 15.5431) (2.2133, 15.5526) (2.2108, 15.5621) (2.2084, 15.5716) (2.2059, 15.5812) (2.2034, 15.5908) (2.2008, 15.6004) (2.1983, 15.61) (2.1957, 15.6197) (2.1931, 15.6294) (2.1905, 15.6391) (2.1879, 15.6488) (2.1852, 15.6585) (2.1825, 15.6683) (2.1798, 15.6781) (2.1771, 15.6879) (2.1743, 15.6978) (2.1715, 15.7076) (2.1687, 15.7175) (2.1659, 15.7274) (2.163, 15.7373) (2.1602, 15.7473) (2.1573, 15.7572) (2.1543, 15.7672) (2.1514, 15.7772) (2.1484, 15.7872) (2.1454, 15.7973) (2.1424, 15.8074) (2.1394, 15.8174) (2.1363, 15.8275) (2.1332, 15.8377) (2.1307, 15.8458) (2.1289, 15.8519) (2.1276, 15.856) (2.127, 15.858) knots 0 0 0 0 0 0 0.00416667 0.00833333 0.0125 0.01666667 0.02083333 0.025 0.02916667 0.03333333 0.0375 0.04166667 0.04583333 0.05 0.05416667 0.05833333 0.0625 0.06666667 0.07083333 0.075 0.07916667 0.08333333 0.0875 0.09166667 0.09583333 0.1 0.10416667 0.10833333 0.1125 0.11666667 0.12083333 0.125 0.12916667 0.13333333 0.1375 0.14166667 0.14583333 0.15 0.15416667 0.15833333 0.1625 0.16666667 0.17083333 0.175 0.17916667 0.18333333 0.1875 0.19166667 0.19583333 0.2 0.20416667 0.20833333 0.2125 0.21666667 0.22083333 0.225 0.22916667 0.23333333 0.2375 0.24166667 0.24583333 0.25 0.25416667 0.25833333 0.2625 0.26666667 0.27083333 0.275 0.27916667 0.28333333 0.2875 0.29166667 0.29583333 0.3 0.30416667 0.30833333 0.3125 0.31666667 0.32083333 0.325 0.32916667 0.33333333 0.3375 0.34166667 0.34583333 0.35 0.35416667 0.35833333 0.3625 0.36666667 0.37083333 0.375 0.37916667 0.38333333 0.3875 0.39166667 0.39583333 0.4 0.40416667 0.40833333 0.4125 0.41666667 0.42083333 0.425 0.42916667 0.43333333 0.4375 0.44166667 0.44583333 0.45 0.45416667 0.45833333 0.4625 0.46666667 0.47083333 0.475 0.47916667 0.48333333 0.4875 0.49166667 0.49583333 0.5 0.50416667 0.50833333 0.5125 0.51666667 0.52083333 0.525 0.52916667 0.53333333 0.5375 0.54166667 0.54583333 0.55 0.55416667 0.55833333 0.5625 0.56666667 0.57083333 0.575 0.57916667 0.58333333 0.5875 0.59166667 0.59583333 0.6 0.60416667 0.60833333 0.6125 0.61666667 0.62083333 0.625 0.62916667 0.63333333 0.6375 0.64166667 0.64583333 0.65 0.65416667 0.65833333 0.6625 0.66666667 0.67083333 0.675 0.67916667 0.68333333 0.6875 0.69166667 0.69583333 0.7 0.70416667 0.70833333 0.7125 0.71666667 0.72083333 0.725 0.72916667 0.73333333 0.7375 0.74166667 0.74583333 0.75 0.75416667 0.75833333 0.7625 0.76666667 0.77083333 0.775 0.77916667 0.78333333 0.7875 0.79166667 0.79583333 0.8 0.80416667 0.80833333 0.8125 0.81666667 0.82083333 0.825 0.82916667 0.83333333 0.8375 0.84166667 0.84583333 0.85 0.85416667 0.85833333 0.8625 0.86666667 0.87083333 0.875 0.87916667 0.88333333 0.8875 0.89166667 0.89583333 0.9 0.90416667 0.90833333 0.9125 0.91666667 0.92083333 0.925 0.92916667 0.93333333 0.9375 0.94166667 0.94583333 0.95 0.95416667 0.95833333 0.9625 0.96666667 0.97083333 0.975 0.97916667 0.98333333 0.9875 0.99166667 0.99583333 1 1 1 1 1 1
  arc A59 (-12.8639, 4.8563) -> (-13.2615, 3.6324) centre (0, 0) ccw
  line L99 (-14.0063, 3.8363) -> (-14.007, 3.8365)
  line L100 (-12.2165, 6.3102) -> (-12.9026, 6.6646)